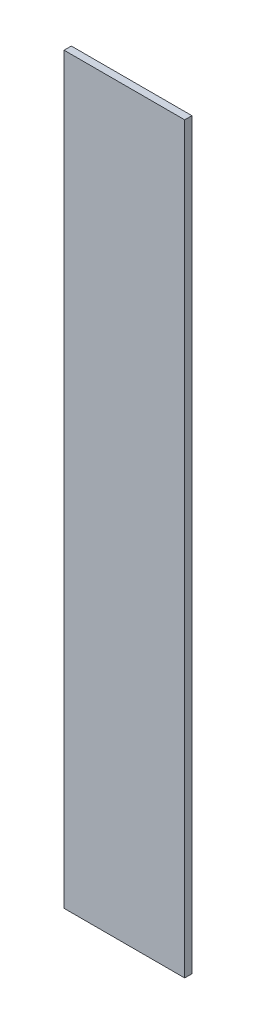
# Autodesk Inventor part: ZAŚLEPKA PRZEDNIA GÓRNY CZARNEJ OBUDOWY STOJAKA
Saved by Autodesk Inventor 2017 SP1 (Build 210196100, 196)
## iProperties
Created: 2020-12-27
Part Number: ZAŚLEPKA PRZEDNIA GÓRNY CZARNEJ OBUDOWY STOJAKA
Material: Tworzywo sztuczne, nieprzezroczyste czarne
Document SubType Name: Modeling
Designer: Napoleon
Mass: 5.4978 g
Surface Area: 82.37 cm^2
Volume: 5.775 cm^3
Density: 0.952 g/cm^3
Appearance: Chropowaty, teksturowany - czarny
Author: Napoleon
Autodesk Inventor part; units mm, degrees
ref_plane "YZ Plane" through (0, 0, 0) normal (1, 0, 0) x (0, 1, 0)
ref_plane "XZ Plane" through (0, 0, 0) normal (0, 1, 0) x (-1, 0, 0)
ref_plane "XY Plane" through (0, 0, 0) normal (0, 0, 1) x (1, 0, 0)
sketch "Szkic1" plane through (0, 0, 0) normal (0, 0, 1) x (1, 0, 0)
  line L0 (-16.5, -97.2419) -> (-16.5, 75.7581) projected
  line L1 (-16.5, 75.7581) -> (16.5, 75.7581) projected
  line L2 (16.5, 75.7581) -> (16.5, -97.2419) projected
  line L3 (-12.5, 75.2581) -> (12.5, 75.2581)
  line L4 (12.5, 75.2581) -> (12.5, -78.7419)
  line L5 (12.5, -78.7419) -> (-12.5, -78.7419)
  line L6 (-12.5, -78.7419) -> (-12.5, 75.2581)
  point P0 (0, 0)
  dimension "d0" = 25
  dimension "d1" = 154
  constraints: 8 end point
  measures "d0" distance of L4.end L5.end
  measures "d1" distance of L3.end L4.end
extrude "Wyciągnięcie proste1" add sketch "Szkic1" against normal blind 1.5
